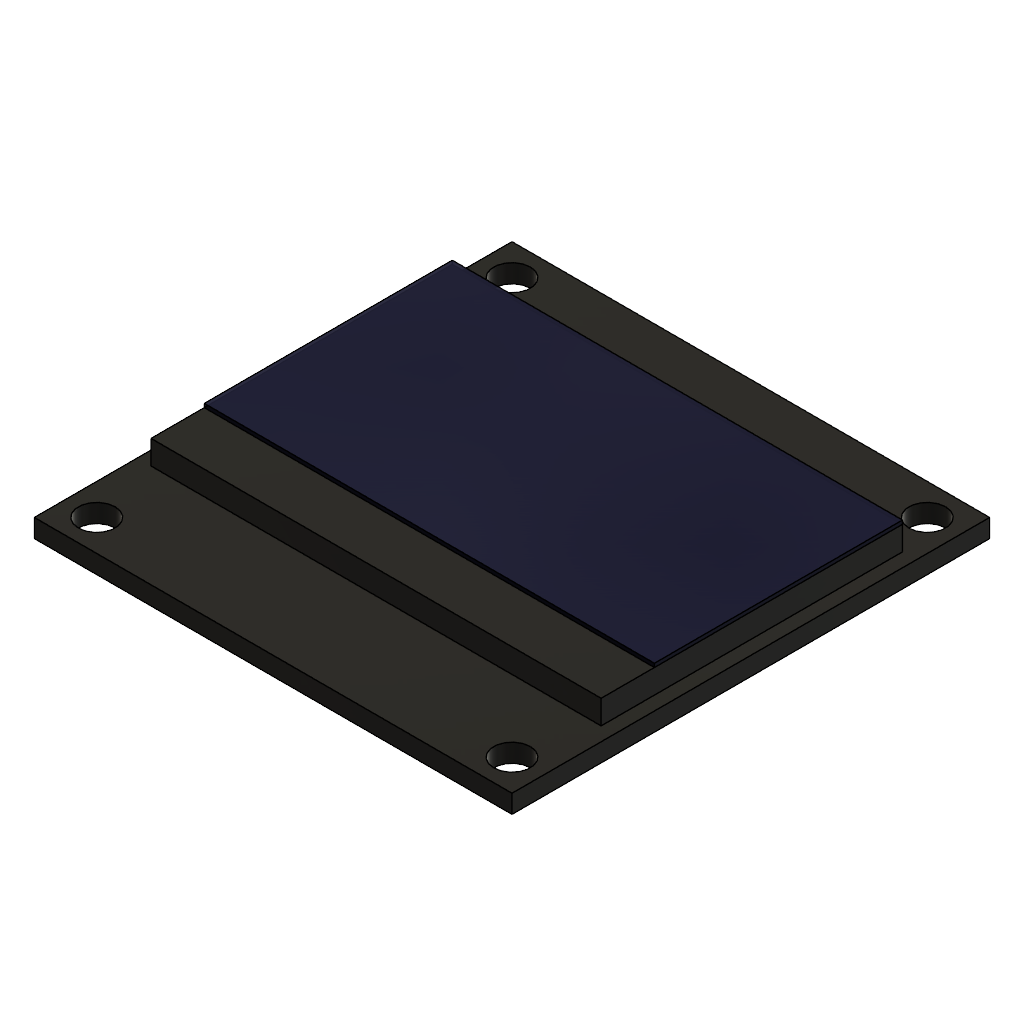
096OLEDModule (Autodesk Fusion 360 design; units mm, degrees)
part number: 2026-08-16-15-52-58-552
Autodesk Fusion 360 part; units mm, degrees
sketch "Sketch1" plane through (0, 0, 0) normal (0, 1, 0) x (1, 0, 0)
  line L0 (13, 13) -> (-13, 13)
  line L1 (-13, 13) -> (-13, -13)
  line L2 (-13, -13) -> (13, -13)
  line L3 (13, -13) -> (13, 13)
  line L4 (13, 13) -> (-13, -13) construction
  line L5 (-13, 13) -> (13, -13) construction
  dimension "d1" = 26
  dimension "d2" = 26
  constraint horizontal L0
  constraint perpendicular L0 L1
  constraint parallel L0 L2
  constraint parallel L1 L3
  constraint coincident L4 origin
  constraint coincident L5 origin
  measures "d1" distance of L1.end L2.end
  measures "d2" distance of L0.end L1.end
extrude "Extrude1" add sketch "Sketch1" along normal blind 1 makes body 1
hole "Hole1" at (-11.3, 1, -11.3) direction (0, -1, 0) diameter 2 depth 3.5 tip angle 118 bodies 1
hole "Hole2" at (11.3, 1, -11.3) direction (0, -1, 0) diameter 2 depth 3.5 tip angle 118 bodies 1
hole "Hole3" at (-11.3, 1, 11.3) direction (0, -1, 0) diameter 2 depth 3.5 tip angle 118 bodies 1
hole "Hole4" at (11.3, 1, 11.3) direction (0, -1, 0) diameter 2 depth 3.5 tip angle 118 bodies 1
sketch "Sketch2" plane through (0, 1, 0) normal (0, 1, 0) x (-1, 0, 0)
  circle A0 centre (-11.3, 11.3) radius 1
  circle A1 centre (11.3, 11.3) radius 1
  circle A2 centre (-11.3, -11.3) radius 1
  circle A3 centre (11.3, -11.3) radius 1
  line L0 (-13, 13) -> (-13, -13)
  line L1 (-13, -13) -> (13, -13)
  line L2 (13, -13) -> (13, 13)
  line L3 (13, 13) -> (-13, 13)
  line L4 (0, -13) -> (0, -9)
  line L5 (0, -9) -> (0, -0.8)
  line L6 (-12.25, -9) -> (12.25, -9)
  line L7 (12.25, -9) -> (12.25, 7.4)
  line L8 (12.25, 7.4) -> (-12.25, 7.4)
  line L9 (-12.25, 7.4) -> (-12.25, -9)
  line L10 (-12.25, -9) -> (12.25, 7.4) construction
  line L11 (12.25, -9) -> (-12.25, 7.4) construction
  point P0 (0, -0.8)
  dimension "d25" = 4
  dimension "d26" = 8.2
  dimension "d27" = 24.5
  dimension "d28" = 16.4
  constraint midpoint L1 L4.start
  constraint perpendicular L1 L4
  constraint parallel L4 L5
  constraint horizontal L6
  constraint perpendicular L6 L7
  constraint parallel L6 L8
  constraint parallel L7 L9
  constraint coincident L10 P0
  constraint coincident L11 P0
  constraint coincident P0 L5.end
  measures "d25" distance of L4.start L4.end
  measures "d26" distance of L4.end P0
  measures "d27" distance of L7.end L8.end
  measures "d28" distance of L6.end L7.end
extrude "Extrude2" add sketch "Sketch2" along normal blind 1.3 separate body contours L6 L7 L8 L9 makes body 2
sketch "Sketch3" plane through (0, 2.3, 0) normal (0, 1, 0) x (-1, 0, 0)
  line L0 (-12.25, 7.4) -> (-12.25, -9)
  line L1 (-12.25, -9) -> (12.25, -9)
  line L2 (12.25, -9) -> (12.25, 7.4)
  line L3 (12.25, 7.4) -> (-12.25, 7.4)
  line L4 (12.25, -9) -> (-12.25, -9)
  line L5 (-12.25, -9) -> (-12.25, 4.5)
  line L6 (-12.25, 4.5) -> (12.25, 4.5)
  line L7 (12.25, 4.5) -> (12.25, -9)
  dimension "d31" = 13.5
  constraint horizontal L4
  constraint vertical L5
  constraint horizontal L6
  constraint vertical L7
  constraint coincident L1.end L2.start
  measures "d31" distance of L1.end L6.end
extrude "Extrude3" add sketch "Sketch3" along normal blind 0.2 separate body contours L0 L1 L2 L4 L5 L6 L7 makes body 3
